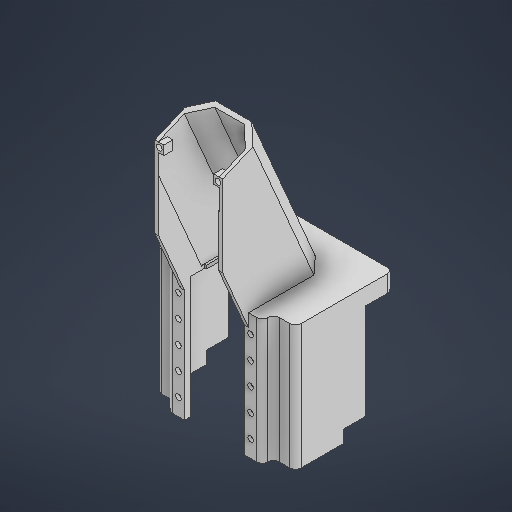
# Autodesk Inventor part: Cover^2
Saved by Autodesk Inventor 2025 (Build 290162000, 162)
## iProperties
Created: 2025-02-14
Part Number: Cover^2
Material: Generic
Document SubType Name: Modeling
Designer: mayhe
Density: 1 g/cm^3
Appearance: Default
Author: mayhe
Autodesk Inventor part; units mm, degrees
ref_plane "YZ Plane" through (0, 0, 0) normal (1, 0, 0) x (0, 1, 0)
ref_plane "XZ Plane" through (0, 0, 0) normal (0, 1, 0) x (-1, 0, 0)
ref_plane "XY Plane" through (0, 0, 0) normal (0, 0, 1) x (1, 0, 0)
sketch "Sketch1" plane through (0, 0, 0) normal (0, 1, 0) x (-1, 0, 0)
  line L0 (58.5, -37.5625) -> (-58.5, -37.5625)
  line L1 (-58.5, -37.5625) -> (-58.5, 37.5625)
  line L2 (-58.5, 37.5625) -> (58.5, 37.5625)
  line L3 (58.5, 37.5625) -> (58.5, -37.5625)
  line L4 (58.5, -37.5625) -> (-58.5, 37.5625) construction
  line L5 (-58.5, -37.5625) -> (58.5, 37.5625) construction
  line L6 (-61.5, -40.5625) -> (61.5, -40.5625)
  line L7 (61.5, -40.5625) -> (61.5, 37.5625)
  line L8 (-61.5, 37.5625) -> (-61.5, -40.5625)
  line L9 (-58.5, 37.5625) -> (-61.5, 37.5625)
  line L10 (58.5, 37.5625) -> (61.5, 37.5625)
  line L11 (-25, 25.0625) -> (25, 25.0625)
  line L12 (25, 25.0625) -> (25, 50.0625)
  line L13 (25, 50.0625) -> (-25, 50.0625)
  line L14 (-25, 50.0625) -> (-25, 25.0625)
  line L15 (-25, 25.0625) -> (25, 50.0625) construction
  line L16 (25, 25.0625) -> (-25, 50.0625) construction
  line L17 (61.5, 37.5625) -> (26.5, 37.5625)
  line L18 (26.5, 37.5625) -> (26.5, 52.5625)
  line L19 (-61.5, 37.5625) -> (-26.5, 37.5625)
  line L20 (-26.5, 37.5625) -> (-26.5, 52.5625)
  line L21 (25, 25.0625) -> (-25, 25.0625)
  line L22 (-25, 25.0625) -> (-25, 10.0625)
  line L23 (-25, 10.0625) -> (25, 10.0625)
  line L24 (25, 10.0625) -> (25, 25.0625)
  circle A0 centre (0, 10.0625) radius 25
  line L25 (61.5, 37.5625) -> (61.5, 45.5625)
  line L26 (61.5, 45.5625) -> (42.25, 45.5625)
  line L27 (42.25, 45.5625) -> (42.25, 55.5625)
  line L28 (42.25, 55.5625) -> (26.5, 55.5625)
  line L29 (26.5, 55.5625) -> (26.5, 52.5625)
  line L30 (-26.5, 52.5625) -> (-26.5, 55.5625)
  line L31 (-26.5, 55.5625) -> (-42.25, 55.5625)
  line L32 (-42.25, 55.5625) -> (-42.25, 45.5625)
  line L33 (-42.25, 45.5625) -> (-61.5, 45.5625)
  line L34 (-61.5, 45.5625) -> (-61.5, 37.5625)
  point P0 (0, 0)
  point P1 (0, 37.5625)
  point P2 (25, 37.5625)
  point P3 (-25, 37.5625)
  point P4 (-26.5, 37.5625)
  point P5 (26.5, 37.5625)
  point P6 (58.5, 37.5625)
  dimension "d1" = 75.125
  dimension "d2" = 3
  dimension "d10" = 50
  dimension "d11" = 25
  dimension "d23" = 3
  dimension "d33" = 50
  dimension "d34" = 15
  dimension "d65" = 8
  dimension "d67" = 10
  dimension "d69" = 15.75
  dimension "d70" = 10
  dimension "d71" = 19.25
  dimension "d72" = 8
  dimension "d85" = 15.75
  dimension "d86" = 19.25
  constraints: 70 end point, 14 perpendicular, 7 parallel, 6 horizontal, 6 midpoint, 1 point on line, 1 vertical, 3 other
  measures "d1" distance between parallel lines of L2 L0
  measures "d2" distance between parallel lines of L0 L6
  measures "d10" distance of L13.end L12.end
  measures "d11" distance of L12.end L11.end
  measures "d23" distance between parallel lines of L3 L7
  measures "d33" distance of L23.end L22.end
  measures "d34" distance of L22.end L21.end
  measures "d65" distance of L7.end L25.end
  measures "d67" distance of L26.end L27.end
  measures "d69" distance of L30.end L31.end
  measures "d70" distance of L31.end L32.end
  measures "d71" distance of L32.end L33.end
  measures "d72" distance of L33.end L8.start
  measures "d85" distance of L27.end L28.end
  measures "d86" distance of L25.end L26.end
extrude "Extrusion1" add sketch "Sketch1" along normal blind 3 contours L3 L10 L7 L6 L8 L9 L1 L0 | L0 L1 L2 L14 L22 A0 L24 L12 L3 | L2 L18 L29 L28 L27 L26 L25 L10 | L9 L34 L33 L32 L31 L30 L20 L2
sketch "Sketch2" plane through (0, 0, 0) normal (0, -1, 0) x (1, 0, 0)
  line L0 (-59.5, 43.5625) -> (-59.5, 20.5625)
  line L1 (-59.5, 20.5625) -> (-61.5, 20.5625)
  line L2 (-61.5, 20.5625) -> (-61.5, 45.5625)
  line L3 (0, 0) -> (0, 37.5625)
  line L4 (59.5, 20.5625) -> (61.5, 20.5625)
  line L5 (-42.25, 55.5625) -> (-26.5, 55.5625)
  line L6 (-26.5, 55.5625) -> (-26.5, 50.5625)
  line L7 (-26.5, 50.5625) -> (-40.25, 50.5625)
  line L8 (-42.25, 45.5625) -> (-61.5, 45.5625)
  line L9 (-59.5, 43.5625) -> (-40.25, 43.5625)
  line L10 (-40.25, 43.5625) -> (-40.25, 50.5625)
  line L11 (-42.25, 45.5625) -> (-42.25, 55.5625) projected
  line L12 (-42.25, 55.5625) -> (-42.25, 45.5625)
  line L13 (59.5, 43.5625) -> (59.5, 20.5625)
  line L14 (59.5, 20.5625) -> (61.5, 20.5625)
  line L15 (61.5, 20.5625) -> (61.5, 45.5625)
  line L16 (42.25, 55.5625) -> (26.5, 55.5625)
  line L17 (26.5, 55.5625) -> (26.5, 50.5625)
  line L18 (26.5, 50.5625) -> (40.25, 50.5625)
  line L19 (42.25, 45.5625) -> (61.5, 45.5625)
  line L20 (59.5, 43.5625) -> (40.25, 43.5625)
  line L21 (40.25, 43.5625) -> (40.25, 50.5625)
  line L22 (42.25, 45.5625) -> (42.25, 55.5625)
  line L23 (42.25, 55.5625) -> (42.25, 45.5625)
  point P0 (0, 25.0625)
  point P1 (-59.5, 53.5625)
  dimension "d6" = 2
  dimension "d27" = 5
  dimension "d76" = 2
  dimension "d77" = 2
  dimension "d78" = 19.25
  dimension "d79" = 19.25
  dimension "d80" = 25
  constraints: 46 end point, 11 symmetric about line, 4 perpendicular, 2 parallel, 1 coincident, 1 collinear, 1 horizontal, 1 vertical, 1 vertical alignment
  measures "d6" distance of L0.end L1.end
  measures "d27" distance of L5.end L6.end
  measures "d76" distance between parallel lines of L11 L10
  measures "d77" distance between parallel lines of L9 L8
  measures "d78" distance of L8.start L2.end
  measures "d79" distance of L0.start L9.end
  measures "d80" distance of L1.end L2.end
extrude "Extrusion2" add sketch "Sketch2" along normal blind 107.5
sketch "Sketch3" plane through (0, 0, 0) normal (0, -1, 0) x (1, 0, 0)
  line L0 (61.5, -40.5625) -> (-61.5, -40.5625) projected
  line L1 (-61.5, -40.5625) -> (61.5, -40.5625)
  line L2 (61.5, -40.5625) -> (61.5, -16.5625)
  line L3 (61.5, -16.5625) -> (56, -16.5625)
  line L4 (56, -16.5625) -> (56, -37.5625)
  line L5 (-61.5, -16.5625) -> (-61.5, -40.5625)
  line L6 (-61.5, -16.5625) -> (-56, -16.5625)
  line L7 (-56, -16.5625) -> (-56, -37.5625)
  line L8 (-56, -37.5625) -> (56, -37.5625)
  line L9 (-59.5, 20.4625) -> (-59.5, -16.5625)
  line L10 (-59.5, -16.5625) -> (-61.5, -16.5625)
  line L11 (61.5, 20.5625) -> (61.5, 55.5625) projected
  line L12 (61.5, 20.5625) -> (59.5, 20.5625)
  line L13 (59.5, 20.5625) -> (59.5, -16.5625)
  line L14 (59.5, -16.5625) -> (61.5, -16.5625)
  line L15 (61.5, -16.5625) -> (61.5, 20.5625)
  line L16 (-61.5, -40.5625) -> (-61.5, 45.5625) projected
  line L17 (-61.5, 20.5625) -> (-61.5, -16.5625)
  line L18 (-61.5, -16.5625) -> (-61.5, -40.5625)
  line L19 (-61.5, 20.5625) -> (-59.5, 20.5625) projected
  line L20 (-61.5, 20.5625) -> (-59.5, 20.5625)
  line L21 (-59.5, 20.5625) -> (-59.5, 20.4625)
  point P0 (0, 0)
  dimension "d12" = 24
  dimension "d13" = 5.5
  dimension "d15" = 90
  dimension "d20" = 5.5
  dimension "d22" = 3
  dimension "d31" = 2
  dimension "d32" = 2
  constraints: 36 end point, 8 perpendicular, 3 collinear, 3 horizontal, 3 point on line, 2 parallel
  measures "d12" distance of L0.start L2.end
  measures "d13" distance of L2.end L3.end
  measures "d15" angle of L4 L3
  measures "d20" distance of L5.start L6.end
  measures "d22" distance between parallel lines of L0 L8
  measures "d31" distance of L9.end L10.end
  measures "d32" distance of L14.end L13.end
extrude "Extrusion3" add sketch "Sketch3" along normal blind 12
fillet "Fillet1" radius 5 16 edges at (56, -6, -37.5625) (-56, -6, -37.5625) (61.5, -4.5, -40.5625) (-61.5, -4.5, -40.5625) (61.5, -52.25, 45.5625) (42.25, -52.25, 45.5625) (42.25, -52.25, 55.5625) (-42.25, -52.25, 55.5625) (-61.5, -52.25, 45.5625) (-42.25, -52.25, 45.5625) (-59.5, -53.75, 43.5625) (-40.25, -53.75, 50.5625) (-40.25, -53.75, 43.5625) (40.25, -53.75, 50.5625) (40.25, -53.75, 43.5625) (59.5, -53.75, 43.5625)
chamfer "Chamfer1" distance 3.5 angle 45 2 edges at (-56, -6, -16.5625) (56, -6, -16.5625)
ref_plane "Work Plane1" through (-42.25, 3, 55.5625) normal (0, 0.9187912, 0.3947439) x (1, 0, 0)
sketch "Sketch4" plane through (-42.25, 3, 55.5625) normal (0, 0.9187912, 0.3947439) x (1, 0, 0)
  line L0 (15.25, 63.1227) -> (69.25, 63.1227)
  line L1 (69.25, 63.1227) -> (69.25, 13.7819)
  ellipse E0 centre (42.25, 41.805) end of major axis (67.25, 41.805) minor radius 22.9698 (67.25, 41.805) -> (17.25, 41.805) ccw
  line L2 (42.25, 41.805) -> (15.25, 63.1227) construction
  line L3 (42.25, 41.805) -> (69.25, 63.1227) construction
  line L4 (12.25, 53.6373) -> (12.25, -4.3627)
  line L5 (72.25, -4.3627) -> (72.25, 53.6373)
  line L6 (72.25, 53.6373) -> (12.25, 53.6373)
  line L7 (15.75, 13.7819) -> (15.25, 13.7819)
  line L8 (15.75, 13.7819) -> (15.75, -4.3627)
  line L9 (67.75, 16.5382) -> (67.75, 0)
  line L10 (69.25, 13.7819) -> (68.75, 13.7819)
  line L11 (68.75, 13.7819) -> (68.75, -4.3627)
  line L12 (12.25, -4.3627) -> (15.75, -4.3627)
  line L13 (68.75, -4.3627) -> (72.25, -4.3627)
  line L14 (15.25, 13.7819) -> (15.25, 63.1227)
  line L15 (12.25, 53.6373) -> (12.25, 67.1227)
  line L16 (12.25, 67.1227) -> (72.25, 67.1227)
  line L17 (72.25, 67.1227) -> (72.25, 53.6373)
  point P0 (42.25, 49.0766)
  point P1 (15.25, 53.6373)
  point P2 (69.25, 53.6373)
  point P3 (42.25, 53.6373)
  point P4 (42.25, 64.7748)
  point P5 (42.25, 67.1227)
  point P6 (42.25, 63.1227)
  dimension "d36" = 54
  dimension "d39" = 58
  dimension "d40" = 3.5
  dimension "d41" = 60
  dimension "d47" = 4
  dimension "d57" = 3
  constraints: 32 end point, 3 midpoint, 3 point on line, 2 vertical alignment, 11 other
  measures "d36" distance of L0.start L0.end
  measures "d39" distance between parallel lines of L6 L12
  measures "d40" distance between parallel lines of L8 L4
  measures "d41" distance of L5.start L4.end
  measures "d47" distance between parallel lines of L0 L16
  measures "d57" distance between parallel lines of L14 L4
extrude "Extrusion4" add sketch "Sketch4" along normal blind 113.55 and the other way blind 55.8 contours L14 L6 L15 L16 L17 L1 L0 E0 | E0 L0 | L14 L7 L8 L12 L4 L6 | L6 L5 L13 L11 L10 L1
chamfer "Chamfer3" distance 14 angle 45 4 edges at (-30, 68.4125, 10.6105) (30, 68.4125, 10.6105) (-27, 67.623, 14.6248) (27, 67.623, 14.6248)
sketch "Sketch8" plane through (30, -8.0519, 55.5625) normal (1, 0, 0) x (0, 0, -1)
  line L0 (-74.8316, 188.6585) -> (-22.8316, 188.6585)
  line L1 (-22.8316, 188.6585) -> (-22.8316, 38.6585)
  line L2 (-22.8316, 38.6585) -> (-74.8316, 38.6585)
  line L3 (-74.8316, 38.6585) -> (-74.8316, 188.6585)
  line L4 (18.0183, -41.9388) -> (-48.8316, 113.6585) projected
  line L5 (-74.8316, 188.6585) -> (-22.8316, 38.6585) construction
  line L6 (-22.8316, 188.6585) -> (-74.8316, 38.6585) construction
  line L7 (5, -11.6378) -> (5, 8.0519) projected
  line L8 (5, 8.0519) -> (5, -11.6378)
  line L9 (83.6985, -13.7204) -> (18.0183, -41.9388) projected
  line L10 (5, -11.6378) -> (18.0183, -41.9388)
  line L11 (18.0183, -41.9388) -> (83.6985, -13.7204)
  line L12 (83.6985, -13.7204) -> (74.3443, 8.0519)
  line L13 (5, 8.0519) -> (74.3443, 8.0519) projected
  line L14 (74.3443, 8.0519) -> (5, 8.0519)
  point P0 (55.5625, 8.0519)
  point P1 (0, 0)
  point P2 (5, -11.6378)
  dimension "d81" = 52
  dimension "d82" = 150
  constraints: 22 end point, 5 perpendicular, 2 midpoint, 2 parallel, 1 horizontal, 1 vertical
  measures "d81" distance of L1.end L2.end
  measures "d82" distance of L0.end L1.end
extrude "Extrusion7" cut sketch "Sketch8" against normal up to surface (60 mm away)
sketch "Sketch9" plane through (0, -12, 0) normal (0, -1, 0) x (1, 0, 0)
  line L0 (0, 0) -> (0, 50)
  line L1 (-61.5, 20.5625) -> (-59.5, 20.5625) projected
  line L2 (-59.5, -16.5625) -> (-59.5, 20.5625) projected
  line L3 (-61.5, 20.5625) -> (-59.5, 20.5625)
  line L4 (-59.5, 20.5625) -> (-59.5, -16.5625)
  line L5 (-59.5, -16.5625) -> (-61.5, -16.5625)
  line L6 (-61.5, -16.5625) -> (-61.5, 20.5625)
  line L7 (61.5, 20.5625) -> (59.5, 20.5625)
  line L8 (59.5, -16.5625) -> (59.5, 20.5625)
  line L9 (61.5, 20.5625) -> (59.5, 20.5625)
  line L10 (59.5, 20.5625) -> (59.5, -16.5625)
  line L11 (59.5, -16.5625) -> (61.5, -16.5625)
  line L12 (61.5, -16.5625) -> (61.5, 20.5625)
  dimension "d92" = 50
  constraints: 22 end point, 5 symmetric about line, 2 parallel, 1 horizontal, 1 perpendicular, 1 vertical
  measures "d92" distance of L0.start L0.end
extrude "Extrusion8" add sketch "Sketch9" along normal blind 95.5
sketch "Sketch10" plane through (0, -107.5, 0) normal (0, -1, 0) x (1, 0, 0)
  line L0 (-59.5, -16.5625) -> (-56, -20.0625) projected
  line L1 (-61.5, 40.5625) -> (-61.5, -16.5625) projected
  line L2 (-59.5, -16.5625) -> (-61.5, -16.5625)
  line L3 (-61.5, -16.5625) -> (-61.5, 3.4375)
  line L4 (-61.5, 3.4375) -> (-59.5, 3.4375)
  line L5 (-59.5, 3.4375) -> (-59.5, -16.5625)
  line L6 (0, 0) -> (0, 17.4625)
  line L7 (59.5, -16.5625) -> (56, -20.0625)
  line L8 (61.5, 40.5625) -> (61.5, -16.5625)
  line L9 (59.5, -16.5625) -> (61.5, -16.5625)
  line L10 (61.5, -16.5625) -> (61.5, 3.4375)
  line L11 (61.5, 3.4375) -> (59.5, 3.4375)
  line L12 (59.5, 3.4375) -> (59.5, -16.5625)
  dimension "d93" = 20
  constraints: 22 end point, 7 symmetric about line, 2 parallel, 2 point on line, 1 horizontal, 1 perpendicular, 1 vertical
  measures "d93" distance of L2.end L3.end
extrude "Extrusion9" cut sketch "Sketch10" against normal blind 11
sketch "Sketch11" plane through (-30, 45.09, 78.3941) normal (0, 0, 1) x (1, 0, 0)
  line L0 (17, 87.1561) -> (43, 87.1561) projected
  line L1 (30, 87.1561) -> (30, 76.2)
  line L2 (0, 71.6871) -> (8, 71.6871)
  line L3 (8, 71.6871) -> (8, 63.6871)
  line L4 (8, 63.6871) -> (0, 63.6871)
  line L5 (0, 63.6871) -> (0, 71.6871)
  line L6 (0, 71.6871) -> (3, 71.6871) projected
  line L7 (60, 71.6871) -> (52, 71.6871)
  line L8 (52, 71.6871) -> (52, 63.6871)
  line L9 (52, 63.6871) -> (60, 63.6871)
  line L10 (60, 63.6871) -> (60, 71.6871)
  line L11 (60, 71.6871) -> (57, 71.6871)
  circle A0 centre (4, 67.6871) radius 2.5
  circle A1 centre (56, 67.6871) radius 2.5
  point P0 (30, -45.09)
  dimension "d96" = 8
  dimension "d97" = 8
  dimension "d98" = 0
  dimension "d111" = 5
  constraints: 20 end point, 7 symmetric about line, 2 centre point, 2 parallel, 1 horizontal, 1 midpoint, 1 perpendicular, 1 vertical, 1 other
  measures "d96" distance of L3.end L4.end
  measures "d97" distance of L2.end L3.end
  measures "d98" distance between parallel lines of L6 L2
  measures "d111" diameter of A0
extrude "Extrusion10" add sketch "Sketch11" against normal blind 8 contours L2 L3 L4 L5 | L10 L9 L8 L7 | A0 | A1
sketch "Sketch12" plane through (26.5, -107.5, 55.5625) normal (0, 0, 1) x (1, 0, 0)
  line L0 (-26.5, 107.5) -> (-26.5, 0.4125)
  line L1 (-53, 0) -> (-63.75, 0) projected
  line L2 (-58.375, 0) -> (-58.375, 110.5)
  line L3 (30, 110.5) -> (-83, 110.5) projected
  line L4 (-58.375, 0) -> (52.125, 0) construction
  circle A0 centre (-58.375, 15) radius 2.5
  circle A1 centre (-58.375, 35) radius 2.5
  circle A2 centre (-58.375, 55) radius 2.5
  circle A3 centre (5.375, 15) radius 2.5
  circle A4 centre (5.375, 35) radius 2.5
  circle A5 centre (5.375, 55) radius 2.5
  circle A6 centre (-58.375, 75) radius 2.5
  circle A7 centre (5.375, 75) radius 2.5
  circle A8 centre (-58.375, 95) radius 2.5
  circle A9 centre (5.375, 95) radius 2.5
  dimension "d101" = 90
  dimension "d102" = 5
  dimension "d103" = 15
  dimension "d106" = 20
  dimension "d116" = 110.5
  constraints: 10 centre point, 6 end point, 5 symmetric about line, 2 midpoint, 2 point on line, 2 vertical, 1 horizontal, 1 perpendicular, 13 other
  measures "d101" angle of L4 L2
  measures "d102" diameter of A0
  measures "d103" distance of point (-58.375, 0) A0.centre
  measures "d106" distance of A0.centre A1.centre
  measures "d116" distance of L2.start L2.end
extrude "Extrusion11" cut sketch "Sketch11" against normal blind 4 contours A0 | A1
extrude "Extrusion12" cut sketch "Sketch12" against normal blind 3
body "Solid1"
